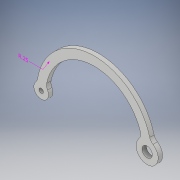
# Autodesk Inventor part: Beta_dummyarm
Saved by Autodesk Inventor 2018 (Build 220112000, 112)
## iProperties
Created: 2017-10-02
Part Number: Beta_dummyarm
Material: Generic
Document SubType Name: Modeling
Designer: rheal
Density: 1 g/cm^3
Appearance: Default
Author: rheal
Autodesk Inventor part; units mm, degrees
ref_plane "YZ Plane" through (0, 0, 0) normal (1, 0, 0) x (0, 1, 0)
ref_plane "XZ Plane" through (0, 0, 0) normal (0, 1, 0) x (-1, 0, 0)
ref_plane "XY Plane" through (0, 0, 0) normal (0, 0, 1) x (1, 0, 0)
sketch "Sketch1" plane through (0, 0, 0) normal (0, 0, 1) x (1, 0, 0)
  line L0 (0, 0) -> (-72, 0) construction
  arc A0 (0, 0) -> (-72, 0) centre (-36, -0.4928) ccw
  arc A1 (1.7364, 9.3676) -> (-74.4764, 5.8972) centre (-36, -0.4928) ccw
  arc A2 (-75.7044, 3.3582) -> (-67.7144, 2.5755) centre (-72, 0) ccw
  arc A3 (-5.6369, 4.9472) -> (3.9444, 6.379) centre (0, 0) ccw
  arc A4 (-2.9997, -0.0411) -> (-3.0003, 0) centre (-36, -0.4928) ccw
  arc A5 (-4.6445, 9.8056) -> (-68.3261, 6.1588) centre (-36, -0.4928) ccw
  arc A6 (-68.9997, 0) -> (-69.0003, -0.0411) centre (-36, -0.4928) ccw
  arc A7 (-68.3261, 6.1588) -> (-67.7144, 2.5755) centre (-63.4287, 5.1511) ccw
  arc A8 (-75.7044, 3.3582) -> (-74.4764, 5.8972) centre (-79.4088, 6.7164) ccw
  arc A9 (-5.6369, 4.9472) -> (-4.6445, 9.8056) centre (-9.3949, 8.2454) ccw
  arc A10 (1.7364, 9.3676) -> (3.9444, 6.379) centre (6.574, 10.6317) ccw
  point P0 (19.05, 139.7)
  point P1 (-67, 0)
  dimension "d79" = 72
  dimension "d83" = 3
  dimension "d85" = 10
  dimension "d86" = 15
  dimension "d87" = 5
  constraints: 22 point on circle, 11 centre point, 8 tangent, 4 coincident, 3 equal radius, 3 point on line, 2 end point, 1 horizontal
  measures "d79" distance of L0.start L0.end
  measures "d83" radial gap between concentric circles of A0 A1
  measures "d85" diameter of A2
  measures "d86" diameter of A3
  measures "d87" radius of A7
extrude "Extrusion1" add sketch "Sketch1" along normal blind 3
sketch "Sketch12" plane through (0, 0, 3) normal (0, 0, 1) x (1, 0, 0)
  circle A0 centre (0, 0) radius 3.5
  arc A1 (-77, 0) -> (-67, 0) centre (-72, 0) ccw projected
  circle A2 centre (-72, 0) radius 1.5
  point P0 (-97.2205, 0)
  dimension "d70" = 7
  dimension "d82" = 3
  constraints: 2 centre point, 2 coincident
  measures "d70" diameter of A0
  measures "d82" diameter of A2
extrude "Extrusion11" cut sketch "Sketch12" against normal blind 5
body "Solid1"
